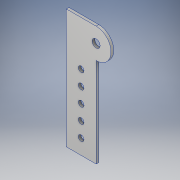
# Autodesk Inventor part: Lifter Bracket
Saved by Autodesk Inventor 2018.3 (Build 223284000, 284)
## iProperties
Created: 2020-01-12
Part Number: Lifter Bracket
Material: Aluminum 6061
Document SubType Name: Modeling
Designer: 22perngrac
Density: 2.7 g/cm^3
Appearance: Aluminum - Flat
Author: 22perngrac
Autodesk Inventor part; units mm, degrees
ref_plane "YZ Plane" through (0, 0, 0) normal (1, 0, 0) x (0, 1, 0)
ref_plane "XZ Plane" through (0, 0, 0) normal (0, 1, 0) x (-1, 0, 0)
ref_plane "XY Plane" through (0, 0, 0) normal (0, 0, 1) x (1, 0, 0)
sketch "Sketch1" plane through (0, 0, 0) normal (0, 0, 1) x (1, 0, 0)
  line L0 (0, 0) -> (25.4, 0)
  line L1 (25.4, 0) -> (25.4, 101.6)
  line L2 (25.4, 101.6) -> (0, 101.6)
  line L3 (0, 101.6) -> (0, 0)
  arc A0 (25.4, 76.2) -> (25.4, 101.6) centre (25.4, 88.9) ccw
  dimension "d0" = 101.6
  dimension "d1" = 25.4
  dimension "d2" = 25.4
  constraints: 8 end point, 2 parallel, 2 point on circle, 2 point on line, 1 centre point, 1 horizontal, 1 perpendicular, 1 tangent
  measures "d0" distance of L2.end L0.start
  measures "d1" distance of L0.start L0.end
  measures "d2" diameter of A0
extrude "Extrusion1" add sketch "Sketch1" along normal blind 2.286
sketch "Sketch3" plane through (0, 0, 2.286) normal (0, 0, 1) x (1, 0, 0)
  line L0 (0, 101.6) -> (0, 0) projected
  line L1 (0, 0) -> (25.4, 0) projected
  line L2 (25.4, 101.6) -> (0, 101.6) projected
  point P0 (12.7, 63.5)
  point P1 (12.7, 50.8)
  point P2 (12.7, 38.1)
  point P3 (12.7, 25.4)
  point P4 (12.7, 12.7)
  dimension "d39" = 38.1
  dimension "d40" = 12.7
  dimension "d43" = 12.7
  constraints: 1 vertical, 4 other
  measures "d39" distance from line of L2 point (12.7, 63.5)
  measures "d40" distance from line of L0 point (12.7, 63.5)
  measures "d43" distance of point (12.7, 63.5) point (12.7, 50.8)
hole "Hole1" at (12.7, 63.5, 2.286) at (12.7, 50.8, 2.286) at (12.7, 38.1, 2.286) at (12.7, 25.4, 2.286) at (12.7, 12.7, 2.286) direction (0, 0, -1) diameter 4.8514 end through all
sketch "Sketch4" plane through (0, 0, 2.286) normal (0, 0, 1) x (1, 0, 0)
  line L0 (25.4, 0) -> (25.4, 76.2) projected
  arc A0 (25.4, 76.2) -> (25.4, 101.6) centre (25.4, 88.9) ccw projected
  point P0 (0, 0)
  constraints: 1 coincident, 1 point on circle
hole "Hole2" at (25.4, 88.9, 2.286) direction (0, 0, -1) diameter 6.7564 end through all clearance for "Flat Head Machine Screw (82)" size "1/4" standard "Ansi Unified Screw Threads"
equation "\"d2\" = d1"
body "Solid1"
